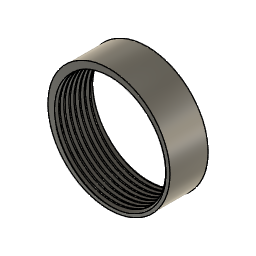
tube_filet_46 (Autodesk Fusion 360 design; units mm, degrees)
Autodesk Fusion 360 part; units mm, degrees
sketch "Esquisse1" plane through (0, 0, 0) normal (0, 1, 0) x (1, 0, 0)
  circle A0 centre (0, 0) radius 24
  circle A1 centre (0.548, 0) radius 23
  dimension "d1" = 48
  dimension "d2" = 46
  constraint coincident A0.centre origin
  measures "d1" diameter of A0
  measures "d2" diameter of A1
extrude "Extrusion1" add sketch "Esquisse1" along normal blind 15
thread "Filetage1" "ISO Metric profile 45.0 M45x2 6H" major diameter 45.2565 minor diameter 43.0224 pitch 2 angle 60 modelled right hand crest width 0.5434 on face at (23.5194, 5, 1.1465) crest through (22.0592, 0.5, 0)
